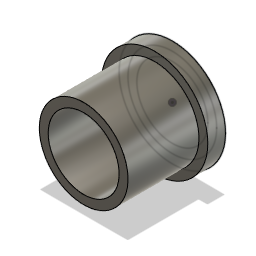
Spool+Lock (Autodesk Fusion 360 design; units mm, degrees)
Autodesk Fusion 360 part; units mm, degrees
sketch "Sketch1" plane through (0, 0, 0) normal (0, 0, 1) x (1, 0, 0)
  circle A0 centre (0, 0) radius 10
  circle A1 centre (0, 0) radius 12.5
  circle A2 centre (0, 0) radius 15
  dimension "d1" = 20
  dimension "d2" = 25
  dimension "d3" = 30
  constraint coincident A0.centre A1.centre
  constraint concentric A0 A2
  measures "d1" diameter of A0
  measures "d2" diameter of A1
  measures "d3" diameter of A2
extrude "Extrude1" add sketch "Sketch1" along normal blind 25 contours A1
extrude "Extrude2" add sketch "Sketch1" along normal blind 5 contours A2
extrude "Extrude3" add sketch "Sketch1" along normal blind 5 contours A0
